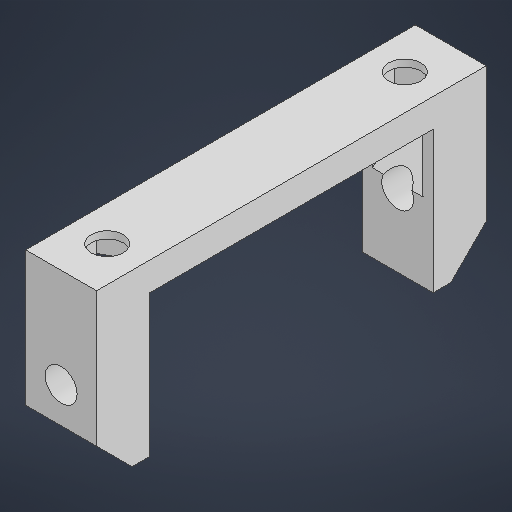
# Autodesk Inventor part: Thread Bearing Bracket
Saved by Autodesk Inventor 2025.1 (Build 291241000, 241)
## iProperties
Created: 2025-02-22
Part Number: Thread Bearing Bracket
Material: Generic
Document SubType Name: Modeling
Designer: jerem
Density: 1 g/cm^3
Appearance: Default
Author: jerem
Autodesk Inventor part; units mm, degrees
ref_plane "YZ Plane" through (0, 0, 0) normal (1, 0, 0) x (0, 1, 0)
ref_plane "XZ Plane" through (0, 0, 0) normal (0, 1, 0) x (-1, 0, 0)
sketch "Sketch1" plane through (0, 0, 0) normal (0, 1, 0) x (-1, 0, 0)
  line L0 (0, 0) -> (10, 0)
  line L1 (10, 0) -> (10, -55)
  line L2 (10, -55) -> (0, -55)
  line L3 (0, -55) -> (0, 0)
  line L4 (5, 0) -> (5, -6.5) construction
  line L5 (5, -6.5) -> (5, -48.5) construction
  circle A0 centre (5, -6.5) radius 2.25
  circle A1 centre (5, -48.5) radius 2.25
  line L6 (5, -27.5) -> (10, -27.5) construction
  line L7 (8.55, -4.4504) -> (8.55, -8.5496)
  line L8 (8.55, -8.5496) -> (5, -10.5992)
  line L9 (5, -10.5992) -> (1.45, -8.5496)
  line L10 (1.45, -8.5496) -> (1.45, -4.4504)
  line L11 (1.45, -4.4504) -> (5, -2.4008)
  line L12 (5, -2.4008) -> (8.55, -4.4504)
  line L13 (5, -44.4008) -> (8.55, -46.4504)
  line L14 (8.55, -46.4504) -> (8.55, -50.5496)
  line L15 (8.55, -50.5496) -> (5, -52.5992)
  line L16 (5, -52.5992) -> (1.45, -50.5496)
  line L17 (1.45, -50.5496) -> (1.45, -46.4504)
  line L18 (1.45, -46.4504) -> (5, -44.4008)
  line L19 (10, -27.5) -> (15, -27.5) construction
  line L20 (15, -27.5) -> (15, -17.5) construction
  line L21 (15, -27.5) -> (15, -37.5) construction
  circle A2 centre (15, -17.5) radius 2.25
  circle A3 centre (15, -37.5) radius 2.25
  line L22 (20, -17.5) -> (20, -37.5)
  line L23 (15, -27.5) -> (20, -27.5) construction
  line L24 (20, -17.5) -> (10, 0)
  line L25 (20, -37.5) -> (10, -55)
  circle A4 centre (15, -17.5) radius 4
  circle A5 centre (15, -37.5) radius 4
  line L26 (0, -27.5) -> (-5, -27.5) construction
  line L27 (-5, -27.5) -> (-5, -17.5) construction
  line L28 (-5, -27.5) -> (-5, -37.5) construction
  circle A6 centre (-5, -17.5) radius 2.25
  circle A7 centre (-5, -37.5) radius 2.25
  line L29 (-10, -17.5) -> (-10, -37.5)
  line L30 (-5, -27.5) -> (-10, -27.5) construction
  line L31 (-10, -17.5) -> (0, 0)
  line L32 (-10, -37.5) -> (0, -55)
  circle A8 centre (-5, -17.5) radius 4
  circle A9 centre (-5, -37.5) radius 4
  dimension "d2" = 10
  dimension "d3" = 55
  dimension "d4" = 7.1
  dimension "d5" = 7.1
  dimension "d6" = 42
  dimension "d7" = 4.5
  dimension "d12" = 20
  dimension "d13" = 4.5
  dimension "d15" = 20
  dimension "d16" = 8
  dimension "d17" = 8
  dimension "d18" = 10
  constraints: 66 end point, 13 coincident, 11 symmetric about line, 10 centre point, 4 midpoint, 4 perpendicular, 3 point on line, 3 vertical, 2 collinear, 2 equal radius, 2 horizontal, 2 parallel, 30 other
  measures "d2" distance of L1.end L2.end
  measures "d3" distance of L0.end L1.end
  measures "d4" distance between parallel lines of L10 L7
  measures "d5" distance between parallel lines of L17 L14
  measures "d6" distance of L5.end A0.centre
  measures "d7" diameter of A0
  measures "d12" distance of L21.end L20.end
  measures "d13" diameter of A2
  measures "d15" distance of L22.start L22.end
  measures "d16" diameter of A4
  measures "d17" diameter of A5
  measures "d18" distance from line of L1.end L22
extrude "Extrusion1" add sketch "Sketch1" along normal blind 4 contours L0 L1 L2 L3 | L7 L8 L9 L10 L11 L12 | L13 L14 L15 L16 L17 L18
extrude "Extrusion2" cut sketch "Sketch1" along normal blind 3 contours L7 L8 L9 L10 L11 L12 | L13 L14 L15 L16 L17 L18
ref_plane "Work Plane1" through (0, 0, -27.5) normal (0, 0, -1) x (-1, 0, 0)
sketch "Sketch2" plane through (0, 0, 0) normal (0, -1, 0) x (1, 0, 0)
  line L0 (-8.55, -4.4504) -> (-5, -2.4008) projected
  line L1 (-5, -2.4008) -> (-1.45, -4.4504) projected
  line L2 (-1.45, -4.4504) -> (-1.45, -8.5496) projected
  line L3 (-1.45, -8.5496) -> (-5, -10.5992) projected
  line L4 (-5, -10.5992) -> (-8.55, -8.5496) projected
  line L5 (-8.55, -8.5496) -> (-8.55, -4.4504) projected
  line L6 (-5, -44.4008) -> (-1.45, -46.4504) projected
  line L7 (-1.45, -46.4504) -> (-1.45, -50.5496) projected
  line L8 (-1.45, -50.5496) -> (-5, -52.5992) projected
  line L9 (-5, -52.5992) -> (-8.55, -50.5496) projected
  line L10 (-8.55, -50.5496) -> (-8.55, -46.4504) projected
  line L11 (-8.55, -46.4504) -> (-5, -44.4008) projected
  line L12 (0, -55) -> (-10, -55) projected
  line L13 (-10, 0) -> (0, 0) projected
  line L14 (4.2857, -7.5) -> (-14.2857, -7.5)
  line L15 (10, -27.5) -> (-20, -27.5) construction
  line L16 (0, 0) -> (0, -55) projected
  line L17 (-10, -55) -> (-10, 0) projected
  point P0 (-10, -7.5)
  point P1 (0, -7.5)
  dimension "d19" = 20
  constraints: 4 end point, 1 horizontal
  measures "d19" distance between parallel lines of L15 L14
extrude "Extrusion3" add sketch "Sketch2" along normal blind 20 contours L5 L14 L17 L13 L16 L2 L1 L0 | L0 L1 L2 L14 L5
extrude "Extrusion4" cut sketch "Sketch1" against normal blind 4 contours A0 | L7 L8 L9 L10 L11 L12
chamfer "Chamfer1" distance 5 angle 45 1 edges at (-5, -4, -7.5)
sketch "Sketch3" plane through (-10, 4, 0) normal (0, 0, 1) x (1, 0, 0)
  line L0 (10, -24) -> (10, 0) projected
  line L1 (0, 0) -> (10, 0) projected
  line L2 (0, -24) -> (0, 0) projected
  line L3 (10, -24) -> (0, -24) projected
  line L4 (5, -24) -> (5, -14) construction
  circle A0 centre (5, -14) radius 2.25
  line L5 (10, -4) -> (0, -4)
  dimension "d27" = 10
  dimension "d28" = 4.5
  constraints: 4 end point, 1 centre point, 1 coincident, 1 midpoint, 1 perpendicular, 1 point on line, 1 vertical
  measures "d27" distance of L4.start L4.end
  measures "d28" diameter of A0
extrude "Extrusion5" cut sketch "Sketch3" against normal through all contours A0
chamfer "Chamfer2" distance 5 angle 45 1 edges at (-5, -20, 0)
mirror "Mirror1" about plane through (0, 0, -27.5) normal (0, 0, -1) of "Extrusion5", "Extrusion3", "Extrusion4", "Chamfer1", "Chamfer2"
equation "\"d5\" = d4"
equation "\"d17\" = d16"
body "Solid1"
